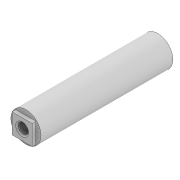
# Autodesk Inventor part: Joint1_Shaft
Saved by Autodesk Inventor 2021 (Build 250183000, 183)
## iProperties
Created: 2020-11-04
Part Number: Joint1_Shaft
Material: Generic
Document SubType Name: Modeling
Designer: Alfred Brauner
Density: 1 g/cm^3
Appearance: Default
Author: Alfred Brauner
Autodesk Inventor part; units mm, degrees
ref_plane "YZ Plane" through (0, 0, 0) normal (1, 0, 0) x (0, 1, 0)
ref_plane "XZ Plane" through (0, 0, 0) normal (0, 1, 0) x (-1, 0, 0)
ref_plane "XY Plane" through (0, 0, 0) normal (0, 0, 1) x (1, 0, 0)
sketch "Sketch1" plane through (0, 0, 0) normal (0, 0, 1) x (1, 0, 0)
  circle A0 centre (0, 0) radius 6
  dimension "d0" = 12
  constraints: 1 centre point, 1 coincident
  measures "d0" diameter of A0
extrude "Extrusion1" add sketch "Sketch1" along normal mid plane 52.5
sketch "Sketch2" plane through (0, 0, 26.25) normal (0, 0, 1) x (1, 0, 0)
  circle A0 centre (0, 0) radius 6
  line L0 (-4, 4) -> (4, 4)
  line L1 (4, 4) -> (4, -4)
  line L2 (4, -4) -> (-4, -4)
  line L3 (-4, -4) -> (-4, 4)
  line L4 (-4, 4) -> (4, -4) construction
  line L5 (4, 4) -> (-4, -4) construction
  dimension "d3" = 12
  dimension "d4" = 8
  dimension "d5" = 8
  constraints: 12 end point, 2 midpoint, 2 parallel, 1 centre point, 1 coincident, 1 horizontal, 1 perpendicular
  measures "d3" diameter of A0
  measures "d4" distance of L1.end L2.end
  measures "d5" distance of L0.end L1.end
extrude "Extrusion2" add sketch "Sketch2" along normal blind 1.5 and the other way blind 34 contours L0 L1 L2 L3
sketch "Sketch6" plane through (0, 0, -26.25) normal (0, 0, -1) x (-1, 0, 0)
  circle A0 centre (0, -4) radius 1.5
  point P0 (0, 0)
  dimension "d28" = 3
  dimension "d29" = 4
  constraints: 1 centre point
  measures "d28" diameter of A0
  measures "d29" distance of A0.centre point (0, 0)
hole "Hole2" at (0, -4, -26.25) direction (0, 0, 1) diameter 3.242 depth 11.8 tip angle 118 counterbore diameter 9 counterbore depth 0 thread size "M4x0.7" class "6H" standard "ISO Metric profile"
sketch "Sketch7" plane through (0, 0, -26.25) normal (0, 0, -1) x (-1, 0, 0)
  point P0 (0, 0)
pattern_circular "Circular Pattern1" count 2 over 360 about axis through (0, 0, 0) along (0, 0, 1) of "Hole2"
sketch "Sketch8" plane through (0, 0, 27.75) normal (0, 0, 1) x (1, 0, 0)
  circle A0 centre (0, 0) radius 1.2628
  constraints: 1 centre point, 1 coincident
hole "Hole3" at (0, 0, 27.75) direction (0, 0, -1) diameter 4.134 depth 14.2 tip angle 118 thread size "M5x0.8" class "6H" standard "ISO Metric profile"
chamfer "Chamfer1" distance 0.5 angle 45 1 edges at (0, 2.067, 27.75)
body "Solid1"
